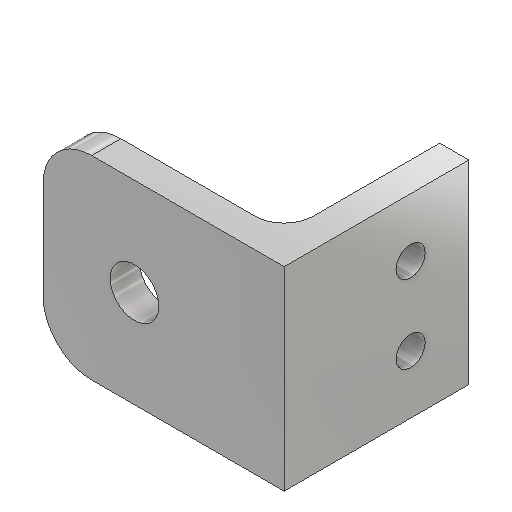
# Autodesk Inventor part: CNCM_ALU_3mm_Y_Axis_Idler_Stiffener_Side
Saved by Autodesk Inventor 2026.1 (Build 301233000, 233)
## iProperties
Created: 2017-05-25
Part Number: CNCM_ALU_3mm_Y_Axis_Idler_Stiffener_Side
Material: Ogólny
Document SubType Name: Modeling
Designer: Andrzej
Density: 1 g/cm^3
Appearance: Aluminium - ciemne
Mass: 2.35312 g
Surface Area: 19.767 cm^2
Volume: 2.35312 cm^3
Author: Andrzej
Autodesk Inventor part; units mm, degrees
ref_plane "YZ Plane" through (0, 0, 0) normal (1, 0, 0) x (0, 1, 0)
ref_plane "XZ Plane" through (0, 0, 0) normal (0, 1, 0) x (-1, 0, 0)
ref_plane "XY Plane" through (0, 0, 0) normal (0, 0, 1) x (1, 0, 0)
sketch "Szkic1" plane through (0, 0, 0) normal (0, 0, 1) x (1, 0, 0)
  line L0 (-11.1928, -2.4042) -> (13.6072, -2.4042)
  line L1 (13.6072, -2.4042) -> (13.6072, 16.5958)
  line L2 (13.6072, 16.5958) -> (10.6072, 16.5958)
  line L3 (10.6072, 16.5958) -> (10.6072, 0.5958)
  line L4 (10.6072, 0.5958) -> (-11.1928, 0.5958)
  line L5 (-11.1928, 0.5958) -> (-11.1928, -2.4042)
  point P0 (0, 0)
  dimension "d0" = 24.8
  dimension "d1" = 19
  dimension "d2" = 3
  dimension "d3" = 16
  constraints: 12 end point, 5 perpendicular, 1 horizontal
  measures "d0" distance of L0.start L0.end
  measures "d1" distance of L0.end L1.end
  measures "d2" distance of L1.end L2.end
  measures "d3" distance of L2.end L3.end
extrude "Wyciągnięcie proste1" add sketch "Szkic1" along normal blind 20
fillet "Zaokrąglenie1" radius 5 2 edges at (-11.1928, -0.9042, 20) (-11.1928, -0.9042, 0)
fillet "Zaokrąglenie2" radius 3 1 edges at (10.6072, 0.5958, 10)
sketch "Szkic2" plane through (-11.1928, 0.5958, 15) normal (0, 1, 0) x (1, 0, 0)
  line L0 (18.8, 15) -> (18.8, -5) projected
  line L1 (18.8, 15) -> (5, 15) projected
  arc A0 (5, 15) -> (0, 10) centre (5, 10) ccw projected
  line L2 (0, 10) -> (0, 0) projected
  arc A1 (0, 0) -> (5, -5) centre (5, 0) ccw projected
  line L3 (18.8, -5) -> (5, -5) projected
  point P0 (11.1928, 15)
  point P1 (9.4, 5)
  dimension "d8" = 10
  dimension "d9" = 18.8
  dimension "d10" = 9.4
  measures "d8" distance from line of L1 point (9.4, 5)
  measures "d9" distance between parallel lines of L0 L2
  measures "d10" distance from line of L2 point (9.4, 5)
hole "Otwór1" at (-1.7928, 0.5958, 10) direction (0, -1, 0) diameter 5 depth 8 tip angle 118
sketch "Szkic3" plane through (10.6072, 16.5958, 0) normal (-1, 0, 0) x (0, 0, 1)
  line L0 (20, -13) -> (0, -13) projected
  line L1 (20, 0) -> (20, -13) projected
  line L2 (0, 0) -> (20, 0) projected
  line L3 (0, 0) -> (0, -13) projected
  point P0 (0, -16.5958)
  point P1 (6, -6)
  point P2 (14, -6)
  dimension "d18" = 6
  dimension "d19" = 6
  dimension "d20" = 6
  dimension "d21" = 6
  measures "d18" distance from line of L2 point (6, -6)
  measures "d19" distance from line of L2 point (14, -6)
  measures "d20" distance from line of L3 point (6, -6)
  measures "d21" distance from line of L1 point (14, -6)
hole "Otwór2" at (10.6072, 10.5958, 6) at (10.6072, 10.5958, 14) direction (1, 0, 0) diameter 3 depth 8 tip angle 118
equation "\"d10\" = 0.5 * d9"
